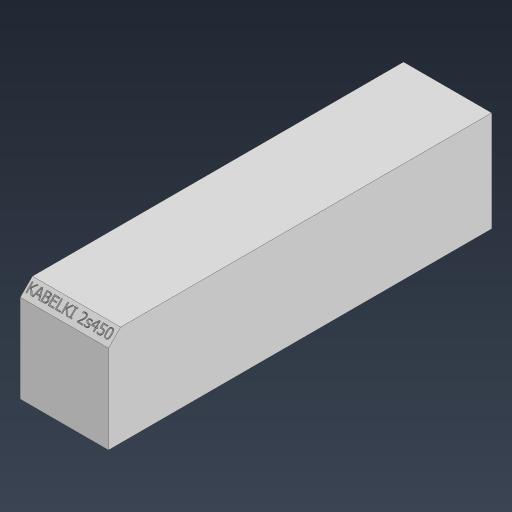
# Autodesk Inventor part: 2s450mah
Saved by Autodesk Inventor 2023 (Build 270158000, 158)
## iProperties
Created: 2026-03-09
Part Number: 2s450mah
Material: Generic
Document SubType Name: Modeling
Designer: szymo
Density: 1 g/cm^3
Appearance: Default
Author: szymo
Autodesk Inventor part; units mm, degrees
ref_plane "YZ Plane" through (0, 0, 0) normal (1, 0, 0) x (0, 1, 0)
ref_plane "XZ Plane" through (0, 0, 0) normal (0, 1, 0) x (-1, 0, 0)
ref_plane "XY Plane" through (0, 0, 0) normal (0, 0, 1) x (1, 0, 0)
sketch "Sketch1" plane through (0, 0, 0) normal (0, 1, 0) x (-1, 0, 0)
  line L0 (0, 0) -> (-14.5, 0)
  line L1 (-14.5, 0) -> (-14.5, -63)
  line L2 (-14.5, -63) -> (0, -63)
  line L3 (0, -63) -> (0, 0)
  dimension "d0" = 14.5
  dimension "d1" = 63
  constraints: 8 end point, 2 parallel, 1 horizontal, 1 perpendicular
  measures "d0" distance of L2.end L1.end
  measures "d1" distance of L0.end L1.end
extrude "Extrusion1" add sketch "Sketch1" along normal blind 16.5
chamfer "Chamfer1" distance 2 angle 45 1 edges at (7.25, 16.5, 0)
sketch "Sketch2" plane through (0, 16.5, -2) normal (0, 0.7071068, 0.7071068) x (1, 0, 0)
  line L0 (0.1727, -0.5129) -> (19.9543, -0.5129) construction
  line L1 (19.9543, -0.5129) -> (19.9543, -3.4313) construction
  line L2 (19.9543, -3.4313) -> (0.1727, -3.4313) construction
  line L3 (0.1727, -3.4313) -> (0.1727, -0.5129) construction
  line L4 (1.4187, -2.0445) -> (1.1597, -2.0445)
  line L5 (1.1597, -2.0445) -> (0.6115, -1.3468)
  line L6 (0.6115, -1.3468) -> (0.524, -1.4452)
  line L7 (0.524, -1.4452) -> (0.524, -2.0445)
  line L8 (0.524, -2.0445) -> (0.3247, -2.0445)
  line L9 (0.3247, -2.0445) -> (0.3247, -0.5445)
  line L10 (0.3247, -0.5445) -> (0.524, -0.5445)
  line L11 (0.524, -0.5445) -> (0.524, -1.2337)
  line L12 (0.524, -1.2337) -> (1.1391, -0.5445)
  line L13 (1.1391, -0.5445) -> (1.3822, -0.5445)
  line L14 (1.3822, -0.5445) -> (0.761, -1.2143)
  line L15 (0.761, -1.2143) -> (1.4187, -2.0445)
  line L16 (1.3761, -2.0445) -> (1.8818, -0.5445)
  line L17 (1.8818, -0.5445) -> (2.1273, -0.5445)
  line L18 (2.1273, -0.5445) -> (2.633, -2.0445)
  line L19 (2.633, -2.0445) -> (2.4227, -2.0445)
  line L20 (2.4227, -2.0445) -> (2.2866, -1.6251)
  line L21 (2.2866, -1.6251) -> (1.714, -1.6251)
  line L22 (1.714, -1.6251) -> (1.5779, -2.0445)
  line L23 (1.5779, -2.0445) -> (1.3761, -2.0445)
  line L24 (2.2319, -1.455) -> (1.9997, -0.7487)
  line L25 (1.9997, -0.7487) -> (1.7687, -1.455)
  line L26 (1.7687, -1.455) -> (2.2319, -1.455)
  spline S0 degree 2 poles (3.7926, -1.5838) (3.7926, -1.6956) (3.7076, -1.867) (3.6371, -1.923) knots 0 0 0 1 2 2 2
  spline S1 degree 2 poles (3.6371, -1.923) (3.552, -1.9886) (3.3587, -2.0445) (3.2055, -2.0445) knots 0 0 0 1 2 2 2
  line L27 (3.2055, -2.0445) -> (2.7752, -2.0445)
  line L28 (2.7752, -2.0445) -> (2.7752, -0.5445)
  line L29 (2.7752, -0.5445) -> (3.1727, -0.5445)
  spline S2 degree 2 poles (3.1727, -0.5445) (3.3332, -0.5445) (3.4936, -0.5652) (3.5666, -0.6053) knots 0 0 0 1 2 2 2
  spline S3 degree 2 poles (3.5666, -0.6053) (3.648, -0.6478) (3.7221, -0.7876) (3.7221, -0.8824) knots 0 0 0 1 2 2 2
  spline S4 degree 2 poles (3.7221, -0.8824) (3.7221, -0.9882) (3.6103, -1.1559) (3.5119, -1.2033) knots 0 0 0 1 2 2 2
  line L30 (3.5119, -1.2033) -> (3.5119, -1.2106)
  spline S5 degree 2 poles (3.5119, -1.2106) (3.6456, -1.2471) (3.7926, -1.4404) (3.7926, -1.5838) knots 0 0 0 1 2 2 2
  spline S6 degree 2 poles (3.5848, -1.5923) (3.5848, -1.5072) (3.5362, -1.3978) (3.4632, -1.3589) knots 0 0 0 1 2 2 2
  spline S7 degree 2 poles (3.4632, -1.3589) (3.4158, -1.3346) (3.304, -1.32) (3.2007, -1.32) knots 0 0 0 1 2 2 2
  line L31 (3.2007, -1.32) -> (2.9746, -1.32)
  line L32 (2.9746, -1.32) -> (2.9746, -1.8743)
  line L33 (2.9746, -1.8743) -> (3.1362, -1.8743)
  spline S8 degree 2 poles (3.1362, -1.8743) (3.2675, -1.8743) (3.4183, -1.85) (3.4766, -1.8111) knots 0 0 0 1 2 2 2
  spline S9 degree 2 poles (3.4766, -1.8111) (3.5325, -1.771) (3.5848, -1.6713) (3.5848, -1.5923) knots 0 0 0 1 2 2 2
  spline S10 degree 2 poles (3.5143, -0.9104) (3.5143, -0.8569) (3.4778, -0.7767) (3.4377, -0.7536) knots 0 0 0 1 2 2 2
  spline S11 degree 2 poles (3.4377, -0.7536) (3.3891, -0.7268) (3.2712, -0.7147) (3.1654, -0.7147) knots 0 0 0 1 2 2 2
  line L34 (3.1654, -0.7147) -> (2.9746, -0.7147)
  line L35 (2.9746, -0.7147) -> (2.9746, -1.1535)
  line L36 (2.9746, -1.1535) -> (3.2007, -1.1535)
  spline S12 degree 2 poles (3.2007, -1.1535) (3.2943, -1.1535) (3.383, -1.1341) (3.4304, -1.1037) knots 0 0 0 1 2 2 2
  spline S13 degree 2 poles (3.4304, -1.1037) (3.4766, -1.0745) (3.5143, -0.9809) (3.5143, -0.9104) knots 0 0 0 1 2 2 2
  line L37 (3.9908, -2.0445) -> (3.9908, -0.5445)
  line L38 (3.9908, -0.5445) -> (4.9292, -0.5445)
  line L39 (4.9292, -0.5445) -> (4.9292, -0.722)
  line L40 (4.9292, -0.722) -> (4.1901, -0.722)
  line L41 (4.1901, -0.722) -> (4.1901, -1.1328)
  line L42 (4.1901, -1.1328) -> (4.8794, -1.1328)
  line L43 (4.8794, -1.1328) -> (4.8794, -1.3103)
  line L44 (4.8794, -1.3103) -> (4.1901, -1.3103)
  line L45 (4.1901, -1.3103) -> (4.1901, -1.867)
  line L46 (4.1901, -1.867) -> (4.9292, -1.867)
  line L47 (4.9292, -1.867) -> (4.9292, -2.0445)
  line L48 (4.9292, -2.0445) -> (3.9908, -2.0445)
  line L49 (6.0171, -2.0445) -> (5.148, -2.0445)
  line L50 (5.148, -2.0445) -> (5.148, -0.5445)
  line L51 (5.148, -0.5445) -> (5.3473, -0.5445)
  line L52 (5.3473, -0.5445) -> (5.3473, -1.867)
  line L53 (5.3473, -1.867) -> (6.0171, -1.867)
  line L54 (6.0171, -1.867) -> (6.0171, -2.0445)
  line L55 (7.2679, -2.0445) -> (7.009, -2.0445)
  line L56 (7.009, -2.0445) -> (6.4608, -1.3468)
  line L57 (6.4608, -1.3468) -> (6.3733, -1.4452)
  line L58 (6.3733, -1.4452) -> (6.3733, -2.0445)
  line L59 (6.3733, -2.0445) -> (6.1739, -2.0445)
  line L60 (6.1739, -2.0445) -> (6.1739, -0.5445)
  line L61 (6.1739, -0.5445) -> (6.3733, -0.5445)
  line L62 (6.3733, -0.5445) -> (6.3733, -1.2337)
  line L63 (6.3733, -1.2337) -> (6.9884, -0.5445)
  line L64 (6.9884, -0.5445) -> (7.2315, -0.5445)
  line L65 (7.2315, -0.5445) -> (6.6103, -1.2143)
  line L66 (6.6103, -1.2143) -> (7.2679, -2.0445)
  line L67 (7.9097, -2.0445) -> (7.3287, -2.0445)
  line L68 (7.3287, -2.0445) -> (7.3287, -1.8914)
  line L69 (7.3287, -1.8914) -> (7.5196, -1.8914)
  line L70 (7.5196, -1.8914) -> (7.5196, -0.6977)
  line L71 (7.5196, -0.6977) -> (7.3287, -0.6977)
  line L72 (7.3287, -0.6977) -> (7.3287, -0.5445)
  line L73 (7.3287, -0.5445) -> (7.9097, -0.5445)
  line L74 (7.9097, -0.5445) -> (7.9097, -0.6977)
  line L75 (7.9097, -0.6977) -> (7.7189, -0.6977)
  line L76 (7.7189, -0.6977) -> (7.7189, -1.8914)
  line L77 (7.7189, -1.8914) -> (7.9097, -1.8914)
  line L78 (7.9097, -1.8914) -> (7.9097, -2.0445)
  line L79 (9.6832, -2.0445) -> (8.7582, -2.0445)
  line L80 (8.7582, -2.0445) -> (8.7582, -1.8318)
  spline S14 degree 2 poles (8.7582, -1.8318) (8.8579, -1.7382) (9.0354, -1.5644) (9.1204, -1.4708) knots 0 0 0 1 2 2 2
  spline S15 degree 2 poles (9.1204, -1.4708) (9.2918, -1.2824) (9.417, -1.0563) (9.417, -0.9359) knots 0 0 0 1 2 2 2
  spline S16 degree 2 poles (9.417, -0.9359) (9.417, -0.8727) (9.3781, -0.7779) (9.3429, -0.7475) knots 0 0 0 1 2 2 2
  spline S17 degree 2 poles (9.3429, -0.7475) (9.3076, -0.7171) (9.2153, -0.6867) (9.1593, -0.6867) knots 0 0 0 1 2 2 2
  spline S18 degree 2 poles (9.1593, -0.6867) (9.1059, -0.6867) (8.9965, -0.7135) (8.9466, -0.7341) knots 0 0 0 1 2 2 2
  spline S19 degree 2 poles (8.9466, -0.7341) (8.9041, -0.7512) (8.8251, -0.7998) (8.8008, -0.8168) knots 0 0 0 1 2 2 2
  line L81 (8.8008, -0.8168) -> (8.7898, -0.8168)
  line L82 (8.7898, -0.8168) -> (8.7898, -0.6029)
  spline S20 degree 2 poles (8.7898, -0.6029) (8.8518, -0.5725) (9.0743, -0.5129) (9.1739, -0.5129) knots 0 0 0 1 2 2 2
  spline S21 degree 2 poles (9.1739, -0.5129) (9.3842, -0.5129) (9.6213, -0.7354) (9.6213, -0.925) knots 0 0 0 1 2 2 2
  spline S22 degree 2 poles (9.6213, -0.925) (9.6213, -1.0137) (9.5799, -1.162) (9.5435, -1.2252) knots 0 0 0 1 2 2 2
  spline S23 degree 2 poles (9.5435, -1.2252) (9.507, -1.2909) (9.4012, -1.4197) (9.3429, -1.4817) knots 0 0 0 1 2 2 2
  spline S24 degree 2 poles (9.3429, -1.4817) (9.2481, -1.585) (9.0159, -1.8063) (8.9466, -1.8707) knots 0 0 0 1 2 2 2
  line L83 (8.9466, -1.8707) -> (9.6832, -1.8707)
  line L84 (9.6832, -1.8707) -> (9.6832, -2.0445)
  spline S25 degree 2 poles (10.2157, -2.0713) (10.1026, -2.0713) (9.9069, -2.0105) (9.8425, -1.9764) knots 0 0 0 1 2 2 2
  line L85 (9.8425, -1.9764) -> (9.8425, -1.7637)
  line L86 (9.8425, -1.7637) -> (9.8522, -1.7637)
  spline S26 degree 2 poles (9.8522, -1.7637) (9.8765, -1.7832) (9.9422, -1.8294) (9.9969, -1.8549) knots 0 0 0 1 2 2 2
  spline S27 degree 2 poles (9.9969, -1.8549) (10.0443, -1.878) (10.161, -1.912) (10.223, -1.912) knots 0 0 0 1 2 2 2
  spline S28 degree 2 poles (10.223, -1.912) (10.2679, -1.912) (10.3713, -1.8914) (10.3956, -1.8743) knots 0 0 0 1 2 2 2
  spline S29 degree 2 poles (10.3956, -1.8743) (10.4308, -1.8512) (10.4624, -1.799) (10.4624, -1.7455) knots 0 0 0 1 2 2 2
  spline S30 degree 2 poles (10.4624, -1.7455) (10.4624, -1.6786) (10.3895, -1.6093) (10.2959, -1.5862) knots 0 0 0 1 2 2 2
  spline S31 degree 2 poles (10.2959, -1.5862) (10.2594, -1.5777) (10.1427, -1.5534) (10.0929, -1.5401) knots 0 0 0 1 2 2 2
  spline S32 degree 2 poles (10.0929, -1.5401) (9.964, -1.5024) (9.8473, -1.3468) (9.8473, -1.2362) knots 0 0 0 1 2 2 2
  spline S33 degree 2 poles (9.8473, -1.2362) (9.8473, -1.083) (10.0771, -0.8922) (10.2667, -0.8922) knots 0 0 0 1 2 2 2
  spline S34 degree 2 poles (10.2667, -0.8922) (10.3603, -0.8922) (10.5499, -0.9384) (10.6144, -0.9736) knots 0 0 0 1 2 2 2
  line L87 (10.6144, -0.9736) -> (10.6144, -1.1766)
  line L88 (10.6144, -1.1766) -> (10.6046, -1.1766)
  spline S35 degree 2 poles (10.6046, -1.1766) (10.5317, -1.1183) (10.3542, -1.0514) (10.2631, -1.0514) knots 0 0 0 1 2 2 2
  spline S36 degree 2 poles (10.2631, -1.0514) (10.1695, -1.0514) (10.0406, -1.1304) (10.0406, -1.2094) knots 0 0 0 1 2 2 2
  spline S37 degree 2 poles (10.0406, -1.2094) (10.0406, -1.2811) (10.1172, -1.3504) (10.2023, -1.3723) knots 0 0 0 1 2 2 2
  spline S38 degree 2 poles (10.2023, -1.3723) (10.2436, -1.3832) (10.3482, -1.4051) (10.4053, -1.4185) knots 0 0 0 1 2 2 2
  spline S39 degree 2 poles (10.4053, -1.4185) (10.5293, -1.4501) (10.6557, -1.5948) (10.6557, -1.72) knots 0 0 0 1 2 2 2
  spline S40 degree 2 poles (10.6557, -1.72) (10.6557, -1.7929) (10.5986, -1.9217) (10.5426, -1.9691) knots 0 0 0 1 2 2 2
  spline S41 degree 2 poles (10.5426, -1.9691) (10.4831, -2.019) (10.3311, -2.0713) (10.2157, -2.0713) knots 0 0 0 1 2 2 2
  line L89 (11.7691, -1.5291) -> (11.5905, -1.5291)
  line L90 (11.5905, -1.5291) -> (11.5905, -2.0445)
  line L91 (11.5905, -2.0445) -> (11.3972, -2.0445)
  line L92 (11.3972, -2.0445) -> (11.3972, -1.5291)
  line L93 (11.3972, -1.5291) -> (10.7347, -1.5291)
  line L94 (10.7347, -1.5291) -> (10.7347, -1.3176)
  line L95 (10.7347, -1.3176) -> (11.4057, -0.5445)
  line L96 (11.4057, -0.5445) -> (11.5905, -0.5445)
  line L97 (11.5905, -0.5445) -> (11.5905, -1.3674)
  line L98 (11.5905, -1.3674) -> (11.7691, -1.3674)
  line L99 (11.7691, -1.3674) -> (11.7691, -1.5291)
  line L100 (11.3972, -1.3674) -> (11.3972, -0.7815)
  line L101 (11.3972, -0.7815) -> (10.8927, -1.3674)
  line L102 (10.8927, -1.3674) -> (11.3972, -1.3674)
  spline S42 degree 2 poles (12.8388, -1.568) (12.8388, -1.6762) (12.7696, -1.861) (12.7063, -1.929) knots 0 0 0 1 2 2 2
  spline S43 degree 2 poles (12.7063, -1.929) (12.6431, -1.9971) (12.4547, -2.0761) (12.338, -2.0761) knots 0 0 0 1 2 2 2
  spline S44 degree 2 poles (12.338, -2.0761) (12.2311, -2.0761) (12.022, -2.0287) (11.9454, -1.991) knots 0 0 0 1 2 2 2
  line L103 (11.9454, -1.991) -> (11.9454, -1.7783)
  line L104 (11.9454, -1.7783) -> (11.96, -1.7783)
  spline S45 degree 2 poles (11.96, -1.7783) (11.9831, -1.7953) (12.0694, -1.8391) (12.1217, -1.8585) knots 0 0 0 1 2 2 2
  spline S46 degree 2 poles (12.1217, -1.8585) (12.1812, -1.8792) (12.2797, -1.9023) (12.3417, -1.9023) knots 0 0 0 1 2 2 2
  spline S47 degree 2 poles (12.3417, -1.9023) (12.4025, -1.9023) (12.5167, -1.8585) (12.558, -1.8111) knots 0 0 0 1 2 2 2
  spline S48 degree 2 poles (12.558, -1.8111) (12.5957, -1.7661) (12.6346, -1.647) (12.6346, -1.5668) knots 0 0 0 1 2 2 2
  spline S49 degree 2 poles (12.6346, -1.5668) (12.6346, -1.4866) (12.5909, -1.3845) (12.5495, -1.3504) knots 0 0 0 1 2 2 2
  spline S50 degree 2 poles (12.5495, -1.3504) (12.507, -1.3127) (12.3806, -1.2811) (12.304, -1.2811) knots 0 0 0 1 2 2 2
  spline S51 degree 2 poles (12.304, -1.2811) (12.2213, -1.2811) (12.0572, -1.3067) (12.0074, -1.3176) knots 0 0 0 1 2 2 2
  line L105 (12.0074, -1.3176) -> (12.0074, -0.5445)
  line L106 (12.0074, -0.5445) -> (12.8303, -0.5445)
  line L107 (12.8303, -0.5445) -> (12.8303, -0.7208)
  line L108 (12.8303, -0.7208) -> (12.2007, -0.7208)
  line L109 (12.2007, -0.7208) -> (12.2007, -1.1207)
  spline S52 degree 2 poles (12.2007, -1.1207) (12.2371, -1.1158) (12.3076, -1.1122) (12.3368, -1.1122) knots 0 0 0 1 2 2 2
  spline S53 degree 2 poles (12.3368, -1.1122) (12.4523, -1.1122) (12.6115, -1.1499) (12.6845, -1.2058) knots 0 0 0 1 2 2 2
  spline S54 degree 2 poles (12.6845, -1.2058) (12.7586, -1.2617) (12.8388, -1.4319) (12.8388, -1.568) knots 0 0 0 1 2 2 2
  spline S55 degree 2 poles (13.9888, -1.2945) (13.9888, -1.6981) (13.7542, -2.0761) (13.5098, -2.0761) knots 0 0 0 1 2 2 2
  spline S56 degree 2 poles (13.5098, -2.0761) (13.2619, -2.0761) (13.0297, -1.6908) (13.0297, -1.2957) knots 0 0 0 1 2 2 2
  spline S57 degree 2 poles (13.0297, -1.2957) (13.0297, -0.8897) (13.2643, -0.5141) (13.5098, -0.5141) knots 0 0 0 1 2 2 2
  spline S58 degree 2 poles (13.5098, -0.5141) (13.7566, -0.5141) (13.9888, -0.9031) (13.9888, -1.2945) knots 0 0 0 1 2 2 2
  spline S59 degree 2 poles (13.7311, -1.7516) (13.7602, -1.6774) (13.7845, -1.4489) (13.7845, -1.2945) knots 0 0 0 1 2 2 2
  spline S60 degree 2 poles (13.7845, -1.2945) (13.7845, -1.1401) (13.7602, -0.9128) (13.7298, -0.8362) knots 0 0 0 1 2 2 2
  spline S61 degree 2 poles (13.7298, -0.8362) (13.6995, -0.7597) (13.5937, -0.6807) (13.5098, -0.6807) knots 0 0 0 1 2 2 2
  spline S62 degree 2 poles (13.5098, -0.6807) (13.426, -0.6807) (13.3178, -0.7597) (13.2862, -0.8387) knots 0 0 0 1 2 2 2
  spline S63 degree 2 poles (13.2862, -0.8387) (13.2558, -0.9153) (13.2339, -1.1486) (13.2339, -1.2957) knots 0 0 0 1 2 2 2
  spline S64 degree 2 poles (13.2339, -1.2957) (13.2339, -1.4538) (13.2533, -1.6653) (13.2849, -1.7479) knots 0 0 0 1 2 2 2
  spline S65 degree 2 poles (13.2849, -1.7479) (13.3141, -1.8257) (13.4223, -1.9096) (13.5098, -1.9096) knots 0 0 0 1 2 2 2
  spline S66 degree 2 poles (13.5098, -1.9096) (13.5925, -1.9096) (13.7007, -1.8306) (13.7311, -1.7516) knots 0 0 0 1 2 2 2
  point P0 (0, -13.0815)
  constraints: 2 other
extrude "Extrusion2" cut sketch "Sketch2" against normal blind 1
body "Solid1"
